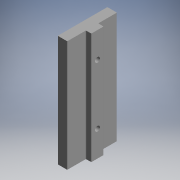
# Autodesk Inventor part: 6825_p2
Saved by Autodesk Inventor 2017.3 (Build 213256000, 256)
## iProperties
Part Number: 6825_p2
Material: Generic
Catalog Web Link: www.cadenas.de
Description: 6725, 6425, 6726, 6426, 6825, 6525, 6826, 6526, 6725-Black, 6425-Black, 6726-Black, 6426-Black, 6825-Black, 6525-Black, 6826-Black, 6526-Black_p2-Double Flange Linear Bearings
Vendor: 8020
Document SubType Name: Modeling
Designer: partserver
Manufacturer: 8020
Mass: 15.5257 g
Surface Area: 63.7711 cm^2
Volume: 15.5257 cm^3
Density: 1 g/cm^3
Appearance: PSOLRGB-191-191-191
Category: PARTsolutions
Company: 8020
Title: 6825_p2
Author: Cadenas PARTsolutions
Comments: Double Flange Linear Bearings
PSOL_IDENT_0: {$CADENAS_DATA\23d-libs\8020\inch\linear_motion\6725_p2.prj},293 {VTYP=3D},{NB=6825_p2},{LINA=6825_p
PSOL_IDENT_1: 2},{NN=6725, 6425, 6726, 6426, 6825, 6525, 6826, 6526, 6725-Black, 6425-Black, 6726-Black, 6426-Blac
PSOL_IDENT_2: k, 6825-Black, 6525-Black, 6826-Black, 6526-Black_p2},{DATE=31.07.2020 09:21:20},{GEOMDATE=19.09.201
PSOL_IDENT_3: 7 12:41:10},{VERSION=},{LINEID=50},{WBVAR=},{WBNUMERIC=}  {NB=6825_p2},{LINA=6825_p2},{KT=DUMMY},{PN=
PSOL_IDENT_4: 6825},{A=1.500},{B=0.500},{C=2.500},{D=0.625},{E=1.250},{F=0.375},{G=4.000},{H=0.750},{J=3.250},{K=1
PSOL_IDENT_5: .250},{L=1.875},{M=1.500},{N=2.812},{P=0.656},{Q=0.000},{R=0.375},{S=0.125},{W=.665},{TH=0.250},{HD=
PSOL_IDENT_6: 0.328},{CS=0.385},{HD1=0.201},{Z=0},{ST=0.190},{PN1=6823},{COLOR=.75,.75,.75}
NB: 6825_p2
NN: 6725, 6425, 6726, 6426, 6825, 6525, 6826, 6526, 6725-Black, 6425-Black, 6726-Black, 6426-Black, 6825-Black, 6525-Black, 6826-Black, 6526-Black_p2
NT: Double Flange Linear Bearings
NBSYN: $PN._p2
LINA: 6825_p2
CATALOG: 80/20
PN: 6825
A: 1.5
B: 0.5
C: 2.5
D: 0.625
E: 1.25
F: 0.375
G: 4
H: 0.75
J: 3.25
K: 1.25
L: 1.875
M: 1.5
N: 2.812
P: 0.656
Q: 0
R: 0.375
S: 0.125
W: .665
ST: 0.19
PN1: 6823
COLOR: .75,.75,.75
SUPPLIER: 8020
ARTICLENO: 6825_p2
BOMINFO: 6825_p2
CREATOR: CADENAS GmbH
Autodesk Inventor part; units mm, degrees
sketch "Sketch_5" plane through (0, 0, 0) normal (0, 0, 1) x (1, 0, 0)
  line L0 (-3.429, 3.556) -> (-3.429, -3.556)
  arc A0 (-3.429, -3.556) -> (-3.048, -3.937) centre (-3.048, -3.556) ccw
  line L1 (-3.048, -3.937) -> (-0.381, -3.937)
  arc A1 (0, -4.318) -> (-0.381, -3.937) centre (-0.381, -4.318) ccw
  line L2 (0, -4.318) -> (0, -15.494)
  arc A2 (0, -15.494) -> (0.381, -15.875) centre (0.381, -15.494) ccw
  line L3 (0.381, -15.875) -> (5.715, -15.875)
  arc A3 (5.715, -15.875) -> (6.096, -15.494) centre (5.715, -15.494) ccw
  line L4 (6.096, -15.494) -> (6.096, 15.494)
  arc A4 (6.096, 15.494) -> (5.715, 15.875) centre (5.715, 15.494) ccw
  line L5 (5.715, 15.875) -> (0.381, 15.875)
  arc A5 (0.381, 15.875) -> (0, 15.494) centre (0.381, 15.494) ccw
  line L6 (0, 15.494) -> (0, 4.318)
  arc A6 (-0.381, 3.937) -> (0, 4.318) centre (-0.381, 4.318) ccw
  line L7 (-0.381, 3.937) -> (-3.048, 3.937)
  arc A7 (-3.048, 3.937) -> (-3.429, 3.556) centre (-3.048, 3.556) ccw
  constraints: 16 end point, 16 point on circle, 8 centre point
extrude "Extrusion1" add sketch "Sketch_5" along normal mid plane 71.12
sketch "Sketch2" plane through (6.096, -15.494, 35.56) normal (1, 0, 0) x (0, 0, -1)
  point P0 (16.51, 15.494)
hole "Hole1" at (6.096, 0, 19.05) direction (-1, 0, 0) diameter 3.175 depth 9.525
sketch "Sketch3" plane through (6.096, -15.494, 35.56) normal (1, 0, 0) x (0, 0, -1)
  point P0 (54.61, 15.494)
hole "Hole2" at (6.096, 0, -19.05) direction (-1, 0, 0) diameter 3.175 depth 9.525
ref_plane "p1_XY" through (6.096, 0, 19.05) normal (1, 0, 0) x (0, 0, -1)
ref_plane "p1_YZ" through (6.096, 0, 19.05) normal (0, 0, -1) x (0, 1, 0)
ref_plane "p1_ZX" through (6.096, 0, 19.05) normal (0, 1, 0) x (1, 0, 0)
body "Solid1"
